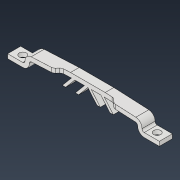
# Autodesk Inventor part: Dribbler Daempfer Oben
Saved by Autodesk Inventor 2022.3 (Build 263350000, 350)
## iProperties
Part Number: Dribbler Daempfer Oben
Material: PVC, hart
Document SubType Name: Modeling
Designer: rYan
Density: 1.29 g/cm^3
Appearance: Glatt - Weiß
Mass: 1.39935 g
Surface Area: 15.5945 cm^2
Volume: 1.08477 cm^3
Author: rYan
Autodesk Inventor part; units mm, degrees
ref_plane "YZ Plane" through (0, 0, 0) normal (1, 0, 0) x (0, 1, 0)
ref_plane "XZ Plane" through (0, 0, 0) normal (0, 1, 0) x (-1, 0, 0)
ref_plane "XY Plane" through (0, 0, 0) normal (0, 0, 1) x (1, 0, 0)
sketch "Skizze1" plane through (0, 0, 0) normal (0, 1, 0) x (-1, 0, 0)
  line L0 (35, 2) -> (28, 2)
  line L1 (35, 2) -> (35, 0)
  line L2 (35, 0) -> (28, 0)
  line L3 (24.1541, 6.1963) -> (8, 7)
  line L4 (24.0547, 4.1988) -> (7.9503, 5)
  line L5 (31, 2) -> (31, 0) construction
  line L6 (8, 7) -> (0, 7)
  line L7 (0, 7) -> (0, 5)
  line L8 (0, 5) -> (7.9503, 5)
  arc A0 (27.0013, 3.05) -> (28, 2) centre (28, 3) ccw
  arc A1 (25.0038, 3.15) -> (28, 0) centre (28, 3) ccw
  arc A2 (25.0038, 3.15) -> (24.0547, 4.1988) centre (24.005, 3.2) ccw
  arc A3 (27.0013, 3.05) -> (24.1541, 6.1963) centre (24.005, 3.2) ccw
  point P0 (0, 0)
  dimension "d0" = 2
  dimension "d1" = 31
  dimension "d2" = 4
  dimension "d5" = 7
  dimension "d6" = 8
  dimension "d7" = 2
  dimension "d8" = 2
  dimension "d26" = 1
  dimension "d27" = 3
  dimension "d28" = 1
  dimension "d29" = 0.2
  constraints: 18 end point, 8 point on circle, 5 tangent, 4 centre point, 4 perpendicular, 4 point on line, 3 coincident, 2 horizontal, 1 parallel, 1 vertical
  measures "d0" distance of L0.start L1.end
  measures "d1" distance from line of point (0, 0) L5
  measures "d2" distance between parallel lines of L1 L5
  measures "d5" distance of point (0, 0) L6.end
  measures "d6" distance of L3.end L6.end
  measures "d7" distance between parallel lines of L4 L3
  measures "d8" distance of L6.end L7.end
  measures "d26" radius of A2
  measures "d27" distance from line of L0.end L5
  measures "d28" radius of A0
  measures "d29" vertical distance of A2.centre A0.centre
extrude "Extrusion1" add sketch "Skizze1" along normal mid plane 6
sketch "Skizze2" plane through (-35, 3, 2) normal (0, 0, 1) x (1, 0, 0)
  line L0 (0, 0) -> (7, 0) projected
  line L1 (0, -6) -> (0, 0) projected
  line L2 (7, -6) -> (0, -6) projected
  line L3 (7, -6) -> (7, 0) projected
  line L4 (35, -7.2) -> (35, 1.2) projected
  line L5 (-7, -3) -> (42, -3) projected
  point P0 (35, -3)
  point P1 (4, -3)
  dimension "d30" = 31
  constraints: 1 point on line
  measures "d30" distance from line of L4 point (4, -3)
hole "Bohrung1" at (-31, 0, 2) direction (0, 0, -1) diameter 3.3 end through all
sketch "Skizze3" plane through (0, 3, 0) normal (0, 1, 0) x (1, 0, 0)
  line L0 (0, -5) -> (-7.9503, -5) projected
  line L1 (-0.0196, -5.3946) -> (-28.1986, -3.9926) projected
  line L2 (0, -5) -> (-4.1955, 0)
  line L3 (-4.1955, 0) -> (-5.762, 0)
  line L4 (-5.762, 0) -> (-1.5665, -5)
  line L5 (0, 1.4) -> (0, -8.4) construction
  point P0 (0, 0)
  point P1 (-28, 0)
  dimension "d19" = 40
  dimension "d20" = 1.2
  constraints: 6 end point, 2 point on line, 1 horizontal, 1 parallel, 1 other
  measures "d19" angle of L5 L2
  measures "d20" distance between parallel lines of L2 L4
extrude "Extrusion2" add sketch "Skizze3" against normal blind 4
pattern_linear "Rechteckige Anordnung1" count 2 spacing 6 along (-1, 0, 0) of "Extrusion2"
mirror "Spiegeln1" about plane through (0, 0, 0) normal (1, 0, 0) of "Extrusion1", "Bohrung1", "Extrusion2", "Rechteckige Anordnung1"
sketch "Skizze4" plane through (-8, -3, 7) normal (0, 0, 1) x (1, 0, 0)
  line L0 (8, 7.2) -> (8, -1.2) construction
  line L1 (0, 0) -> (16, 0) construction
  line L2 (-6, 0) -> (-4, 2)
  line L3 (-4, 2) -> (20, 2)
  line L4 (20, 2) -> (22, 0)
  line L5 (22, 0) -> (-6, 0)
  point P0 (8, 3)
  dimension "d31" = 2
  dimension "d32" = 24
  dimension "d33" = 45
  constraints: 8 end point, 1 collinear, 1 horizontal, 1 parallel, 1 other
  measures "d31" distance between parallel lines of L3 L1
  measures "d32" distance of L2.end L3.end
  measures "d33" angle of L5 L2
extrude "Extrusion3" cut sketch "Skizze4" against normal through all
fillet "Rundung1" radius 2 4 edges at (-14, -3, 5.7002) (-12, -1, 5.7998) (12, -1, 5.7998) (14, -3, 5.7002)
